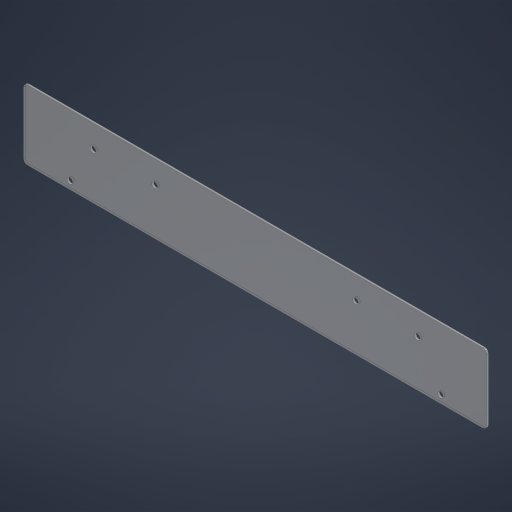
# Autodesk Inventor part: wedge
Saved by Autodesk Inventor 2024 (Build 280153000, 153)
## iProperties
Created: 2023-11-18
Part Number: wedge
Material: Polycarbonate, Clear
Document SubType Name: Modeling
Designer: macbook
Density: 1.2 g/cm^3
Appearance: Polycarbonate - Clear(1)
Author: macbook
Autodesk Inventor part; units mm, degrees
ref_plane "YZ Plane" through (0, 0, 0) normal (1, 0, 0) x (0, 1, 0)
ref_plane "XZ Plane" through (0, 0, 0) normal (0, 1, 0) x (-1, 0, 0)
ref_plane "XY Plane" through (0, 0, 0) normal (0, 0, 1) x (1, 0, 0)
sketch "Sketch1" plane through (0, 0, 0) normal (0, 0, 1) x (1, 0, 0)
  line L0 (0, 0) -> (-381, 0)
  line L1 (-381, -3.175) -> (-381, 47.625)
  line L2 (-377.825, 50.8) -> (-3.175, 50.8)
  line L3 (0, 47.625) -> (0, 0)
  line L4 (-381, 0) -> (-381, -6.35)
  line L5 (-377.825, -6.35) -> (-3.175, -6.35)
  line L6 (0, -3.175) -> (0, 0)
  arc A0 (-381, -3.175) -> (-377.825, -6.35) centre (-377.825, -3.175) ccw
  arc A1 (-377.825, 50.8) -> (-381, 47.625) centre (-377.825, 47.625) ccw
  arc A2 (0, 47.625) -> (-3.175, 50.8) centre (-3.175, 47.625) ccw
  arc A3 (-3.175, -6.35) -> (0, -3.175) centre (-3.175, -3.175) ccw
  point P0 (-381, 50.8)
  point P1 (0, 50.8)
  point P2 (0, -6.35)
  dimension "d1" = 50.8
  dimension "d7" = 6.35
  dimension "d19" = 3.175
  dimension "d20" = 3.175
  constraints: 14 end point, 8 point on circle, 8 point on line, 8 tangent, 4 centre point, 3 perpendicular, 2 equal radius, 2 horizontal, 2 vertical
  measures "d1" distance of L0.end point (-381, 50.8)
  measures "d7" distance of L0.end L4.end
  measures "d19" radius of A0
  measures "d20" radius of A3
extrude "Extrusion1" add sketch "Sketch1" along normal blind 1.5875
sketch "Sketch2" plane through (0, 0, 1.5875) normal (0, 0, 1) x (1, 0, 0)
  line L0 (-381, 50.8) -> (-323.85, 50.8)
  line L1 (-323.85, 50.8) -> (-273.05, 50.8)
  line L2 (-273.05, 50.8) -> (-273.05, 31.75)
  line L3 (-381, 0) -> (-342.9, 0)
  line L4 (-323.85, 50.8) -> (-323.85, 31.75)
  line L5 (-190.5, 50.8) -> (-190.5, -6.35)
  line L6 (0, 50.8) -> (-57.15, 50.8)
  line L7 (-57.15, 50.8) -> (-107.95, 50.8)
  line L8 (-107.95, 50.8) -> (-107.95, 31.75)
  line L9 (0, 0) -> (-38.1, 0)
  line L10 (-57.15, 50.8) -> (-57.15, 31.75)
  dimension "d4" = 57.15
  dimension "d5" = 50.8
  dimension "d6" = 19.05
  dimension "d11" = 38.1
  constraints: 22 end point, 10 symmetric about line, 6 coincident, 2 vertical, 1 horizontal
  measures "d4" distance of L0.start L0.end
  measures "d5" distance of L0.end L1.end
  measures "d6" distance of L1.end L2.end
  measures "d11" distance of L3.start L3.end
hole "Hole1" at (-323.85, 31.75, 1.5875) at (-273.05, 31.75, 1.5875) at (-342.9, 0, 1.5875) at (-107.95, 31.75, 1.5875) at (-57.15, 31.75, 1.5875) at (-38.1, 0, 1.5875) direction (0, 0, -1) diameter 4.7625 end through all
body "Solid1"
